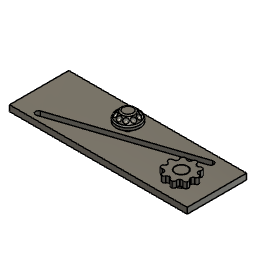
Assembly Modeling (Autodesk Fusion 360 design; units mm, degrees)
Autodesk Fusion 360 part; units mm, degrees
note: some values were not read from the file. Set by a fixed rule: which sketch regions a step uses.
sketch "Sketch1" plane through (0, 0, 0) normal (0, 1, 0) x (1, 0, 0) in component "Base"
  line L0 (75, -25) -> (-75, -25)
  line L1 (-75, -25) -> (-75, 25)
  line L2 (-75, 25) -> (75, 25)
  line L3 (75, 25) -> (75, -25)
  line L4 (75, -25) -> (-75, 25) construction
  line L5 (-75, -25) -> (75, 25) construction
  line L6 (-55.8901, -21.2653) -> (53.2085, 15.1009)
  arc A0 (53.2085, 15.1009) -> (51.6273, 19.8443) centre (52.4179, 17.4726) ccw
  line L7 (51.6273, 19.8443) -> (-57.4713, -16.5219)
  arc A1 (-57.4713, -16.5219) -> (-55.8901, -21.2653) centre (-56.6807, -18.8936) ccw
  line L8 (-56.6807, -18.8936) -> (52.4179, 17.4726) construction
  circle A2 centre (55, -10) radius 5
  dimension "d1" = 150
  dimension "d2" = 50
  dimension "d3" = 5
  dimension "d4" = 115
  dimension "d21" = 10
  dimension "d22" = 15
  dimension "d23" = 20
  constraint horizontal L0
  constraint perpendicular L0 L1
  constraint parallel L0 L2
  constraint parallel L1 L3
  constraint coincident L4 origin
  constraint coincident L5 origin
  constraint tangent L6 A0
  constraint tangent A0 L7
  constraint parallel L6 L7
  constraint tangent L7 A1
  constraint tangent L6 A1
  constraint coincident L5 A0.centre
  constraint parallel L5 L8
  measures "d1" distance of L1.end L2.end
  measures "d2" distance of L0.end L1.end
  measures "d3" diameter of A0
  measures "d4" distance of A1.centre A0.centre
  measures "d21" diameter of A2
  measures "d22" distance of L0 A2.centre
  measures "d23" distance of L3 A2.centre
extrude "Extrude1" add sketch "Sketch1" along normal blind 5 contours L0 L1 L2 L3 | A2 makes body 1 in component "Base"
extrude "Extrude2" add sketch "Sketch1" along normal blind 15 contours A2 bodies 1 in component "Base"
sketch "Sketch1 (2)" plane through (0, 0, 0) normal (1, 0, 0) x (0, 0, -1) in component "Knob"
  line L0 (0, 0) -> (0, 26)
  line L1 (0, 26) -> (5, 26)
  line L2 (5, 26) -> (10, 21)
  line L3 (10, 21) -> (10, 18)
  line L4 (10, 18) -> (2.5, 18)
  line L5 (2.5, 18) -> (2.5, 12)
  line L6 (2.5, 12) -> (0, 12)
  dimension "d7" = 5
  dimension "d8" = 6
  dimension "d9" = 20
  dimension "d10" = 14
  dimension "d11" = 12
  dimension "d12" = 45
  dimension "d13" = 5
  constraint coincident L0.start origin
  constraint vertical L0
  constraint perpendicular L0 L1
  constraint perpendicular L1 L3
  constraint perpendicular L3 L4
  constraint perpendicular L4 L5
  constraint coincident L0 L6.end
  constraint perpendicular L0 L6
  measures "d8" distance of L4.end L5.end
  measures "d10" distance of L1 L6
  measures "d11" distance of L0.start L6
  measures "d12" angle of L1 L2
  measures "d13" horizontal distance of L1.end L2.end
revolve "Revolve1" add sketch "Sketch1 (2)" angle 360 about axis through (0, 0, 0) along (0, 1, 0) separate body makes body 2 in component "Knob"
sketch "Sketch2" plane through (0, 0, 0) normal (1, 0, 0) x (0, 0, -1) in component "Knob"
  line L0 (10, 21) -> (5, 26)
  line L1 (-5, 26) -> (-10, 21)
  line L2 (7.5, 23.5) -> (7.5, 25.5)
  circle A0 centre (7.5, 23.5) radius 2
  line L3 (7.5, 23.5) -> (7.5, 21.5)
  dimension "d15" = 2
  constraint midpoint L0 L2.start
  constraint vertical L2
  constraint coincident L2.start A0.centre
  constraint coincident L2.end A0
  constraint coincident A0 L3.end
  constraint parallel L2 L3
  measures "d15" distance of L2.start L2.end
revolve "Revolve2" cut sketch "Sketch2" angle 360 about axis through (0, 23.5, -7.5) along (0, 1, 0) contours L0 A0 L3 | L0 L2 A0 picked at (8.3772, 22.4997) picked at (8.7995, 23.7827) bodies 2 in component "Knob"
pattern_circular "C-Pattern1" count 10 over 360 about axis through (0, 26, 0) along (0, -1, 0) of "Revolve2" in component "Knob"
fillet "Fillet1" radius 2 2 edges at (-4.6616, 26, -1.8081) (-9.3233, 21, -3.6162) on bodies 2 in component "Knob"
sketch "Sketch1 (3)" plane through (0, 5, 0) normal (0, 1, 0) x (-1, 0, 0) in component "Gear"
  circle A0 centre (-55, 10) radius 5
  arc A1 (57.4713, 16.5219) -> (55.8901, 21.2653) centre (56.6807, 18.8936) ccw
  line L0 (57.4713, 16.5219) -> (-51.6273, -19.8443)
  arc A2 (-53.2085, -15.1009) -> (-51.6273, -19.8443) centre (-52.4179, -17.4726) ccw
  line L1 (-53.2085, -15.1009) -> (55.8901, 21.2653)
  line L2 (-75, -25) -> (75, -25)
  line L3 (75, -25) -> (75, 25)
  line L4 (75, 25) -> (-75, 25)
  line L5 (-75, 25) -> (-75, -25)
  circle A3 centre (-55, 10) radius 5
  circle A4 centre (-55, 10) radius 5.25
  circle A5 centre (-55, 10) radius 10
  line L6 (-57, 3) -> (-53, 3)
  line L7 (-53, 3) -> (-53, -3)
  line L8 (-53, -3) -> (-57, -3)
  line L9 (-57, -3) -> (-57, 3)
  line L10 (-57, 3) -> (-53, -3) construction
  line L11 (-53, 3) -> (-57, -3) construction
  point P0 (-55, 0)
  dimension "d26" = 10.5
  dimension "d27" = 20
  dimension "d28" = 4
  dimension "d29" = 6
  constraint concentric A3 A4
  constraint concentric A3 A5
  constraint horizontal L6
  constraint perpendicular L6 L7
  constraint parallel L6 L8
  constraint parallel L7 L9
  constraint coincident L10 P0
  constraint coincident L11 P0
  constraint coincident A5 P0
  constraint vertical A0.centre P0
  measures "d26" diameter of A4
  measures "d27" diameter of A5
  measures "d28" distance of L7.end L8.end
  measures "d29" distance of L6.end L7.end
extrude "Extrude1'" add sketch "Sketch1 (3)" along normal blind 5 from surface at 5 separate body contours A5 L6 L7 L9 | A5 L6 L7 L9 makes body 3 in component "Gear"
extrude "Extrude2'" add sketch "Sketch1 (3)" along normal blind 5 from surface at 5 contours A5 L7 L8 L9 bodies 3 in component "Gear"
fillet "Fillet1'" radius 2 4 edges at (53, 12.5, 0.202) (57, 12.5, 0.202) (57, 12.5, -3) (53, 12.5, -3) on bodies 3 in component "Gear"
pattern_circular "C-Pattern1'" count 9 over 360 about axis through (55, 15, 10) along (0, 1, 0) of "Extrude2'", "Fillet1'" in component "Gear"
component "Base" placed x (1, 0, 0) y (0, 1, 0) z (0, 0, 1) at (0, 0, 0)
component "Knob" placed x (1, 0, 0) y (0, 1, 0) z (0, 0, 1) at (0, 0, 0)
component "Gear" placed x (1, 0, 0) y (0, 1, 0) z (0, 0, 1) at (0, 0, 0)
